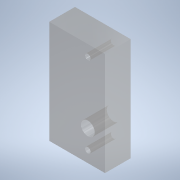
# Autodesk Inventor part: Top
Saved by Autodesk Inventor 2020 (Build 240168000, 168)
## iProperties
Created: 2019-02-07
Part Number: Top
Material: 유리
Document SubType Name: Modeling
Designer: Jeong Ji Hoon
Density: 2.18 g/cm^3
Appearance: 연회색 반사
Author: Jeong Ji Hoon
Autodesk Inventor part; units mm, degrees
ref_plane "YZ Plane" through (0, 0, 0) normal (1, 0, 0) x (0, 1, 0)
ref_plane "XZ Plane" through (0, 0, 0) normal (0, 1, 0) x (-1, 0, 0)
ref_plane "XY Plane" through (0, 0, 0) normal (0, 0, 1) x (1, 0, 0)
sketch "스케치1" plane through (0, 0, 0) normal (0, 0, 1) x (1, 0, 0)
  line L0 (0, 0) -> (4, 0)
  line L1 (4, 0) -> (4, 12)
  line L2 (4, 12) -> (0, 12)
  line L3 (0, 12) -> (0, 0)
  dimension "d0" = 4
  dimension "d1" = 12
  constraints: 8 end point, 2 parallel, 1 horizontal, 1 perpendicular
  measures "d0" distance of L2.end L1.end
  measures "d1" distance of L1.end L0.end
extrude "돌출1" add sketch "스케치1" along normal blind 3
sketch "스케치2" plane through (0, 0, 3) normal (0, 0, 1) x (1, 0, 0)
  line L0 (4, 12) -> (0, 12) construction
  line L1 (2, 12) -> (2, 0) construction
  line L2 (0, 0) -> (4, 0) construction
  line L3 (0, 7) -> (4, 7)
  line L4 (4, 7) -> (4, 6)
  line L5 (4, 6) -> (0, 6)
  line L6 (0, 6) -> (0, 7)
  line L7 (4, 0) -> (4, 12) projected
  line L8 (0, 12) -> (0, 0) projected
  point P0 (2, 7.7)
  point P1 (2, 3.5)
  point P2 (2, 1.3)
  point P3 (2, 7.7)
  point P4 (2, 10.7)
  dimension "d7" = 1
  dimension "d8" = 5
  dimension "d9" = 4.3
  dimension "d45" = 1.3
  dimension "d51" = 4.2
  dimension "d52" = 2.2
  dimension "d54" = 0
  dimension "d55" = 1.3
  constraints: 10 end point, 4 point on line, 2 collinear, 2 midpoint, 2 parallel, 1 coincident, 1 horizontal, 1 perpendicular
  measures "d7" distance between parallel lines of L5 L3
  measures "d8" distance between parallel lines of L0 L3
  measures "d9" distance from line of L0 point (2, 7.7)
  measures "d45" distance from line of point (2, 1.3) L2
  measures "d51" distance of point (2, 3.5) point (2, 7.7)
  measures "d52" distance of point (2, 1.3) point (2, 3.5)
  measures "d54" distance of point (2, 7.7) point (2, 7.7)
  measures "d55" distance from line of point (2, 10.7) L0
hole "구멍2" at (2, 3.5, 3) direction (0, 0, -1) diameter 1.6 end through all
hole "구멍3" at (2, 1.3, 3) at (2, 10.7, 3) direction (0, 0, -1) diameter 0.65 end through all
sketch "스케치3" plane through (0, 0, 3) normal (0, 0, 1) x (1, 0, 0)
  circle A0 centre (2, 1.3) radius 0.325 projected
  circle A1 centre (2, 10.7) radius 0.325 projected
  circle A2 centre (2, 3.5) radius 0.8 projected
  line L0 (0, 0) -> (4, 0) projected
  line L1 (4, 0) -> (4, 12) projected
  line L2 (4, 12) -> (0, 12) projected
  line L3 (0, 12) -> (0, 0) projected
  line L4 (0, 0) -> (-2.5, 0)
  line L5 (-2.5, 0) -> (-2.5, 12)
  line L6 (-2.5, 12) -> (0, 12)
  line L7 (0, 12) -> (0, 0)
  dimension "d57" = 2.5
  constraints: 8 end point, 2 parallel, 1 collinear, 1 horizontal, 1 perpendicular
  measures "d57" distance of L5.end L6.end
extrude "돌출3" add sketch "스케치3" against normal up to surface (3 mm away) contours L4 L5 L6 L3
equation "\"G23_M\" = 0.67"
equation "\"G23_F\" = 0.65"
